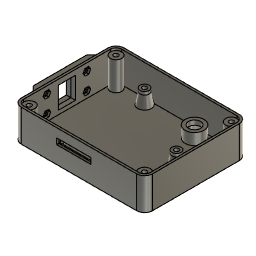
MainCaseBottom (Autodesk Fusion 360 design; units mm, degrees)
Autodesk Fusion 360 part; units mm, degrees
sketch "Skizze1" plane through (0, 0, 0) normal (0, 0, 1) x (1, 0, 0)
  line L0 (0, 0) -> (115, 0)
  line L1 (115, 0) -> (115, 90)
  line L2 (115, 90) -> (0, 90)
  line L3 (0, 90) -> (0, 0)
  dimension "d1" = 115
  dimension "d2" = 90
  constraint horizontal L0
  constraint vertical L1
  constraint horizontal L2
  constraint vertical L3
  constraint coincident L0.start L3.end
  measures "d1" distance of L0.start L0.end
  measures "d2" distance of L0.end L1.end
extrude "Extrusion1" add sketch "Skizze1" along normal blind 28 makes body 1
sketch "Skizze3" plane through (0, 0, 28) normal (0, 0, 1) x (-1, 0, 0)
  line L0 (0, -90) -> (0, 0)
  line L1 (0, 0) -> (-115, 0)
  line L2 (-115, 0) -> (-115, -90)
  line L3 (-115, -90) -> (0, -90)
  line L4 (-2, -88) -> (-113, -88)
  line L5 (-113, -88) -> (-113, -2)
  line L6 (-113, -2) -> (-2, -2)
  line L7 (-2, -2) -> (-2, -88)
  dimension "d7" = 2
  dimension "d8" = 2
  dimension "d9" = 2
  dimension "d10" = 2
  constraint horizontal L4
  constraint vertical L5
  constraint horizontal L6
  constraint vertical L7
  measures "d7" distance of L2 L5
  measures "d8" distance of L3 L4
  measures "d9" distance of L0 L7
  measures "d10" distance of L1 L6
extrude "Extrusion2" cut sketch "Skizze3" against normal blind 27 contours L4 L5 L6 L7 bodies 1
fillet "Abrundung2" radius 5 4 edges at (113, 88, 14.5) (2, 88, 14.5) (2, 2, 14.5) (113, 2, 14.5) on bodies 1
fillet "Abrundung3" radius 7 4 edges at (0, 90, 14) (115, 90, 14) (115, 0, 14) (0, 0, 14) on bodies 1
sketch "Skizze4" plane through (0, 0, 1) normal (0, 0, 1) x (-1, 0, 0)
  arc A0 (-108, -2) -> (-113, -7) centre (-108, -7) ccw
  line L0 (-113, -7) -> (-113, -83)
  arc A1 (-113, -83) -> (-108, -88) centre (-108, -83) ccw
  line L1 (-108, -88) -> (-7, -88)
  arc A2 (-7, -88) -> (-2, -83) centre (-7, -83) ccw
  line L2 (-2, -83) -> (-2, -7)
  arc A3 (-2, -7) -> (-7, -2) centre (-7, -7) ccw
  line L3 (-7, -2) -> (-108, -2)
  arc A4 (-113, -83) -> (-108, -88) centre (-108, -83) ccw
  arc A5 (-108, -2) -> (-113, -7) centre (-108, -7) ccw
  arc A6 (-2, -7) -> (-7, -2) centre (-7, -7) ccw
  arc A7 (-7, -88) -> (-2, -83) centre (-7, -83) ccw
  circle A8 centre (-108, -83) radius 5
  circle A9 centre (-108, -7) radius 5
  circle A10 centre (-7, -7) radius 5
  circle A11 centre (-7, -83) radius 5
  constraint concentric A4 A8
  constraint coincident L0.end A8
  constraint concentric A5 A9
  constraint coincident A0.end A9
  constraint concentric A3 A10
  constraint coincident A3.end A10
  constraint concentric A7 A11
  constraint coincident L1.end A11
extrude "Extrusion3" add sketch "Skizze4" along normal blind 25 contours A0 A5 A9 | A3 A6 A10 | A1 A4 A8 | A2 A7 A11 bodies 1
sketch "Skizze6" plane through (0, 0, 26) normal (0, 0, 1) x (-1, 0, 0)
  arc A0 (-113, -83) -> (-108, -88) centre (-108, -83) ccw
  arc A1 (-108, -88) -> (-113, -83) centre (-108, -83) ccw
  arc A2 (-108, -2) -> (-113, -7) centre (-108, -7) ccw
  arc A3 (-113, -7) -> (-108, -2) centre (-108, -7) ccw
  arc A4 (-7, -88) -> (-2, -83) centre (-7, -83) ccw
  arc A5 (-2, -83) -> (-7, -88) centre (-7, -83) ccw
  arc A6 (-7, -2) -> (-2, -7) centre (-7, -7) ccw
  arc A7 (-2, -7) -> (-7, -2) centre (-7, -7) ccw
  point P0 (-7, -83)
  point P1 (-108, -83)
  point P2 (-108, -7)
  point P3 (-7, -7)
  constraint coincident P0 A4.centre
  constraint coincident P1 A0.centre
  constraint coincident P2 A2.centre
  constraint coincident P3 A6.centre
hole "Bohrung1" at (108, 83, 26) at (108, 7, 26) at (7, 7, 26) at (7, 83, 26) direction (0, 0, -1) diameter 4 depth 20 tip angle 180 bodies 1
sketch "Skizze9" plane through (0, 0, 0) normal (-1, 0, 0) x (0, -1, 0)
  line L0 (-7, 0) -> (-7, 28)
  line L1 (-7, 28) -> (-83, 28)
  line L2 (-83, 28) -> (-83, 0)
  line L3 (-83, 0) -> (-7, 0)
  line L4 (-72.5, 28) -> (-17.5, 28)
  line L5 (-17.5, 28) -> (-17.5, 0)
  line L6 (-17.5, 0) -> (-72.5, 0)
  line L7 (-72.5, 0) -> (-72.5, 28)
  dimension "d39" = 55
  dimension "d40" = 17.5
  constraint horizontal L4
  constraint vertical L5
  constraint horizontal L6
  constraint vertical L7
  constraint coincident L3 L5.end
  measures "d39" distance of L5.end L6.end
  measures "d40" distance of origin L5
extrude "Extrusion5" add sketch "Skizze9" along normal blind 4 separate body contours L1 L3 L4 L5 L6 L7 makes body 2
chamfer "Fase1" distance 4 angle 45 2 edges at (-4, 17.5, 14) (-4, 72.5, 14) on bodies 2
sketch "Skizze10" plane through (-4, 0, 0) normal (-1, 0, 0) x (0, -1, 0)
  line L0 (-68.5, 28) -> (-68.5, 0)
  line L1 (-68.5, 0) -> (-21.5, 0)
  line L2 (-21.5, 0) -> (-21.5, 28)
  line L3 (-21.5, 28) -> (-68.5, 28)
  line L4 (-50.5, 21.5) -> (-39.5, 21.5)
  line L5 (-39.5, 21.5) -> (-39.5, 6.5)
  line L6 (-39.5, 6.5) -> (-50.5, 6.5)
  line L7 (-50.5, 6.5) -> (-50.5, 21.5)
  dimension "d44" = 11
  dimension "d45" = 15
  dimension "d46" = 18
  dimension "d47" = 18
  dimension "d48" = 6.5
  dimension "d49" = 6.5
  constraint horizontal L4
  constraint vertical L5
  constraint horizontal L6
  constraint vertical L7
  measures "d44" distance of L5.end L6.end
  measures "d45" distance of L4.end L5.end
  measures "d46" distance of L2 L5
  measures "d47" distance of L0 L7
  measures "d48" distance of L1 L6
  measures "d49" distance of L3 L4
extrude "Extrusion6" cut sketch "Skizze10" against normal blind 10 contours L4 L5 L6 L7 bodies 1 2
sketch "Skizze11" plane through (-4, 0, 0) normal (-1, 0, 0) x (0, -1, 0)
  line L0 (-39.5, 21.5) -> (-39.5, 6.5)
  line L1 (-39.5, 6.5) -> (-50.5, 6.5)
  line L2 (-50.5, 6.5) -> (-50.5, 21.5)
  line L3 (-50.5, 21.5) -> (-39.5, 21.5)
  line L4 (-68.5, 28) -> (-68.5, 0)
  line L5 (-68.5, 0) -> (-21.5, 0)
  line L6 (-21.5, 0) -> (-21.5, 28)
  line L7 (-21.5, 28) -> (-68.5, 28)
  point P0 (-62.5, 21.5)
  point P1 (-27.5, 21.5)
  point P2 (-27.5, 6.5)
  point P3 (-62.5, 6.5)
  dimension "d52" = 35
  dimension "d53" = 35
  dimension "d54" = 15
  dimension "d55" = 15
  dimension "d56" = 6
  dimension "d57" = 6
  dimension "d58" = 6.5
  dimension "d59" = 6.5
  constraint horizontal P0 P1
  constraint vertical P0 P3
  measures "d52" distance of P2 P3
  measures "d53" horizontal distance of P0 P1
  measures "d54" distance of P1 P2
  measures "d55" vertical distance of P0 P3
  measures "d56" distance of L4 P0
  measures "d57" distance of L6 P1
  measures "d58" distance of L7 P1
  measures "d59" distance of L5 P2
hole "Bohrung3" at (-4, 27.5, 21.5) at (-4, 27.5, 6.5) at (-4, 62.5, 6.5) at (-4, 62.5, 21.5) direction (1, 0, 0) diameter 3.5 depth 12 tip angle 180 bodies 1 2
sketch "Skizze12" plane through (2, 0, 0) normal (1, 0, 0) x (0, 1, 0)
  circle A0 centre (62.5, 6.5) radius 1.75
  circle A1 centre (27.5, 21.5) radius 1.75
  circle A2 centre (27.5, 6.5) radius 1.75
  circle A3 centre (62.5, 21.5) radius 1.75
  line L0 (39.5, 6.5) -> (39.5, 21.5)
  line L1 (39.5, 21.5) -> (50.5, 21.5)
  line L2 (50.5, 21.5) -> (50.5, 6.5)
  line L3 (50.5, 6.5) -> (39.5, 6.5)
  line L4 (7, 26) -> (7, 1)
  line L5 (7, 1) -> (83, 1)
  line L6 (83, 1) -> (83, 26)
  line L7 (83, 26) -> (83, 28)
  line L8 (83, 28) -> (7, 28)
  line L9 (7, 28) -> (7, 26)
  circle A4 centre (62.5, 21.5) radius 1.75
  circle A5 centre (62.5, 6.5) radius 1.75
  circle A6 centre (27.5, 6.5) radius 1.75
  circle A7 centre (27.5, 21.5) radius 1.75
  line L10 (30.8486, 21.5) -> (29.1743, 24.4)
  line L11 (29.1743, 24.4) -> (25.8257, 24.4)
  line L12 (25.8257, 24.4) -> (24.1514, 21.5)
  line L13 (24.1514, 21.5) -> (25.8257, 18.6)
  line L14 (25.8257, 18.6) -> (29.1743, 18.6)
  line L15 (29.1743, 18.6) -> (30.8486, 21.5)
  line L16 (65.8486, 21.5) -> (64.1743, 24.4)
  line L17 (64.1743, 24.4) -> (60.8257, 24.4)
  line L18 (60.8257, 24.4) -> (59.1514, 21.5)
  line L19 (59.1514, 21.5) -> (60.8257, 18.6)
  line L20 (60.8257, 18.6) -> (64.1743, 18.6)
  line L21 (64.1743, 18.6) -> (65.8486, 21.5)
  line L22 (65.8486, 6.5) -> (64.1743, 9.4)
  line L23 (64.1743, 9.4) -> (60.8257, 9.4)
  line L24 (60.8257, 9.4) -> (59.1514, 6.5)
  line L25 (59.1514, 6.5) -> (60.8257, 3.6)
  line L26 (60.8257, 3.6) -> (64.1743, 3.6)
  line L27 (64.1743, 3.6) -> (65.8486, 6.5)
  line L28 (30.8486, 6.5) -> (29.1743, 9.4)
  line L29 (29.1743, 9.4) -> (25.8257, 9.4)
  line L30 (25.8257, 9.4) -> (24.1514, 6.5)
  line L31 (24.1514, 6.5) -> (25.8257, 3.6)
  line L32 (25.8257, 3.6) -> (29.1743, 3.6)
  line L33 (29.1743, 3.6) -> (30.8486, 6.5)
  point P0 (27.5, 21.5)
  point P1 (62.5, 21.5)
  point P2 (62.5, 6.5)
  point P3 (27.5, 6.5)
  dimension "d63" = 5.8
  dimension "d64" = 5.8
  dimension "d65" = 5.8
  dimension "d66" = 5.8
  constraint coincident P0 A1.centre
  constraint coincident P1 A3.centre
  constraint coincident P2 A0.centre
  constraint coincident A2.centre A6.centre
  constraint horizontal L14
  constraint horizontal L20
  constraint horizontal L26
  constraint horizontal L32
  measures "d63" distance of L11 L14
  measures "d64" distance of L17 L20
  measures "d65" distance of L23 L26
  measures "d66" distance of L29 L32
extrude "Extrusion7" cut sketch "Skizze12" against normal blind 3 contours L10 L11 L12 L13 L14 L15 | L16 L17 L18 L19 L20 L21 | L22 L23 L24 L25 L26 L27 | L28 L29 L30 L31 L32 L33 bodies 1 2
sketch "Skizze13" plane through (0, 0, 1) normal (0, 0, 1) x (-1, 0, 0)
  arc A0 (-113, -7) -> (-108, -2) centre (-108, -7) ccw
  line L0 (-113, -7) -> (-113, -83)
  arc A1 (-108, -88) -> (-113, -83) centre (-108, -83) ccw
  line L1 (-108, -88) -> (-7, -88)
  arc A2 (-2, -83) -> (-7, -88) centre (-7, -83) ccw
  line L2 (-2, -83) -> (-2, -7)
  arc A3 (-7, -2) -> (-2, -7) centre (-7, -7) ccw
  line L3 (-7, -2) -> (-108, -2)
  circle A4 centre (-79.3, -79.5) radius 8.25
  circle A5 centre (-79.3, -8.5) radius 8.25
  line L4 (-7, 0) -> (-108, 0)
  dimension "d69" = 16.5
  dimension "d70" = 16.5
  dimension "d71" = 71
  dimension "d72" = 8.5
  dimension "d86" = 79.3
  constraint vertical A4.centre A5.centre
  measures "d69" diameter of A4
  measures "d70" diameter of A5
  measures "d71" distance of A4.centre A5.centre
  measures "d72" distance of A5.centre L4
  measures "d86" horizontal distance of origin A5.centre
extrude "Extrusion8" cut sketch "Skizze13" along normal mid plane 20 contours L3 A5 | L3 A5 | A4 bodies 1
sketch "Skizze16" plane through (0, 0, 0) normal (0, 0, 1) x (1, 0, 0)
  circle A0 centre (79.3, 79.5) radius 8.25
  circle A1 centre (79.3, 8.5) radius 8.25
extrude "Extrusion10" add sketch "Skizze16" along normal blind 11 separate body makes body 3 at (87.5397, 79.0888, 7.3333) makes body 4 at (87.5397, 8.0888, 7.3333)
sketch "Skizze17" plane through (0, 0, 11) normal (0, 0, 1) x (-1, 0, 0)
  circle A0 centre (-79.3, -8.5) radius 8.25
  circle A1 centre (-79.3, -79.5) radius 8.25
  circle A2 centre (-79.3, -8.5) radius 8.25
  point P0 (-79.3, -79.5)
  point P1 (-79.3, -8.5)
  constraint coincident P0 A1.centre
  constraint coincident P1 A0.centre
hole "Bohrung5" at (79.3, 79.5, 11) at (79.3, 8.5, 11) direction (0, 0, -1) diameter 10.5 depth 22 tip angle 180 bodies 3 4
chamfer "Fase2" distance 2 distance2 7 1 edges at (74.4053, 6.6015, 0) measured on face at (86.5144, 7.9594, 0) on bodies 3 4
chamfer "Fase2" distance 2 distance2 7 1 edges at (74.4053, 77.6015, 0) measured on face at (86.5144, 78.9594, 0) on bodies 3 4
sketch "Skizze18" plane through (0, 0, 1) normal (0, 0, 1) x (-1, 0, 0)
  arc A0 (-84.3806, -2) -> (-74.2194, -2) centre (-79.3, -8.5) ccw
  line L0 (-84.3806, -2) -> (-108, -2)
  arc A1 (-113, -7) -> (-108, -2) centre (-108, -7) ccw
  line L1 (-113, -7) -> (-113, -83)
  arc A2 (-108, -88) -> (-113, -83) centre (-108, -83) ccw
  line L2 (-108, -88) -> (-7, -88)
  arc A3 (-2, -83) -> (-7, -88) centre (-7, -83) ccw
  line L3 (-2, -83) -> (-2, -7)
  arc A4 (-7, -2) -> (-2, -7) centre (-7, -7) ccw
  line L4 (-7, -2) -> (-74.2194, -2)
  circle A5 centre (-79.3, -79.5) radius 8.25
  circle A6 centre (-32, -83) radius 4
  circle A7 centre (-32, -7) radius 4
  circle A8 centre (-93, -50) radius 4
  line L5 (-108, -90) -> (-7, -90)
  line L6 (-7, 0) -> (-108, 0)
  line L7 (-71.3655, -10.7597) -> (-72.4783, -3.8603)
  arc A9 (-71.3655, -10.7597) -> (-72.4783, -3.8603) centre (-70, -7) ccw
  dimension "d96" = 8
  dimension "d97" = 8
  dimension "d98" = 8
  dimension "d99" = 8
  dimension "d100" = 76
  dimension "d101" = 7
  dimension "d102" = 7
  dimension "d103" = 32
  dimension "d104" = 38
  dimension "d105" = 61
  dimension "d106" = 43
  constraint vertical A6.centre A7.centre
  constraint horizontal A7.centre A9.centre
  constraint coincident A0 L7.start
  constraint coincident A0 L7.end
  measures "d96" diameter of A6
  measures "d97" diameter of A7
  measures "d98" diameter of A9
  measures "d99" diameter of A8
  measures "d100" distance of A6.centre A7.centre
  measures "d101" distance of A6.centre L5
  measures "d102" distance of A7.centre L6
  measures "d103" horizontal distance of origin A7.centre
  measures "d104" horizontal distance of A7.centre A9.centre
  measures "d105" horizontal distance of A7.centre A8.centre
  measures "d106" vertical distance of A7.centre A8.centre
extrude "Extrusion11" add sketch "Skizze18" along normal blind 12.7 contours A0 A9 | A6 | A7 | A8 bodies 1 4
sketch "Skizze19" plane through (0, 0, 13.7) normal (0, 0, 1) x (-1, 0, 0)
  arc A0 (-71.3655, -10.7597) -> (-72.4783, -3.8603) centre (-70, -7) ccw
  arc A1 (-71.3655, -10.7597) -> (-72.4783, -3.8603) centre (-79.3, -8.5) ccw
  arc A2 (-71.3655, -10.7597) -> (-72.4783, -3.8603) centre (-70, -7) ccw
  circle A3 centre (-70, -7) radius 4
  constraint concentric A2 A3
  constraint coincident A0.start A3
extrude "Extrusion12" add sketch "Skizze19" against normal blind 4.7 contours A1 A3 bodies 1
sketch "Skizze20" plane through (0, 0, 13.7) normal (0, 0, 1) x (-1, 0, 0)
  circle A0 centre (-93, -50) radius 4
  circle A1 centre (-32, -83) radius 4
  circle A2 centre (-70, -7) radius 4
  circle A3 centre (-32, -7) radius 4
  point P0 (-32, -83)
  point P1 (-93, -50)
  point P2 (-70, -7)
  point P3 (-32, -7)
  constraint coincident P0 A1.centre
  constraint coincident A0.centre P1
  constraint coincident P2 A2.centre
  constraint coincident P3 A3.centre
hole "Bohrung6" at (32, 83, 13.7) at (93, 50, 13.7) at (70, 7, 13.7) at (32, 7, 13.7) direction (0, 0, -1) diameter 4 depth 12 tip angle 180 bodies 1
sketch "Skizze21" plane through (0, 0, 0) normal (0, -1, 0) x (1, 0, 0)
  line L0 (7, 28) -> (7, 0)
  line L1 (7, 0) -> (108, 0)
  line L2 (108, 0) -> (108, 28)
  line L3 (108, 28) -> (7, 28)
  line L4 (39, 19.3) -> (67, 19.3)
  line L5 (67, 19.3) -> (67, 16.1)
  line L6 (67, 16.1) -> (39, 16.1)
  line L7 (39, 16.1) -> (39, 19.3)
  dimension "d117" = 16.1
  dimension "d118" = 3.2
  dimension "d119" = 39
  dimension "d120" = 67
  constraint horizontal L4
  constraint vertical L5
  constraint horizontal L6
  constraint vertical L7
  measures "d117" vertical distance of origin L6.end
  measures "d118" distance of L4.end L5.end
  measures "d119" horizontal distance of origin L6.end
  measures "d120" horizontal distance of origin L5.end
extrude "Extrusion13" cut sketch "Skizze21" against normal blind 3 contours L4 L5 L6 L7 bodies 1
chamfer "Fase4" distance 1 angle 45 4 edges at (53, 0, 16.1) (39, 0, 17.7) (53, 0, 19.3) (67, 0, 17.7) on bodies 1
chamfer "Fase5" distance 2 distance2 10 1 edges at (35.7293, 81.5535, 1) measured on face at (47.0263, 54.35, 1) on bodies 1
chamfer "Fase5" distance 2 distance2 10 1 edges at (96.7293, 48.5535, 1) measured on face at (47.0263, 54.35, 1) on bodies 1
chamfer "Fase5" distance 2 distance2 10 1 edges at (66.051, 6.3631, 1) measured on face at (47.0263, 54.35, 1) on bodies 1
chamfer "Fase5" distance 2 distance2 10 1 edges at (35.7293, 5.5535, 1) measured on face at (47.0263, 54.35, 1) on bodies 1
chamfer "Fase6" distance 2 angle 45 4 edges at (2, 45, 6.5) (2, 50.5, 14) (2, 45, 21.5) (2, 39.5, 14) on bodies 1
equation "d3 = 29 mm - 1 mm"
equation "d46 = d47"
equation "d48 = d49"
equation "d56 = d57"
equation "d58 = d59"
equation "d72 = d73"
equation "d73 = 8.50 mm"
equation "d101 = d102"
equation "d112 = 8 mm - 12.7 mm"
equation "d117 = ( 29 / 2 ) * 1 mm + 1.6 mm"
equation "d119 = 32 mm + 7 mm"
equation "d120 = 32 mm + 35 mm"
